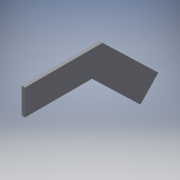
# Autodesk Inventor part: lower gusset
Saved by Autodesk Inventor 2016 (Build 200138000, 138)
## iProperties
Created: 2016-02-23
Part Number: lower gusset
Material: Aluminum 6061
Document SubType Name: Modeling
Designer: gus
Density: 2.7 g/cm^3
Appearance: Aluminum - Flat
Author: gus
Autodesk Inventor part; units mm, degrees
ref_plane "YZ Plane" through (0, 0, 0) normal (1, 0, 0) x (0, 1, 0)
ref_plane "XZ Plane" through (0, 0, 0) normal (0, 1, 0) x (-1, 0, 0)
ref_plane "XY Plane" through (0, 0, 0) normal (0, 0, 1) x (1, 0, 0)
sketch "Sketch1" plane through (0, 0, 0) normal (1, 0, 0) x (0, 1, 0)
  line L0 (0, 0) -> (0, -101.6)
  line L1 (0, -101.6) -> (-52.8555, -156.4884)
  line L2 (-25.4, 2.4125) -> (-25.4, -91.3586)
  line L3 (-25.4, -91.3586) -> (-71.1516, -138.8699)
  line L4 (-52.8555, -156.4884) -> (-71.1516, -138.8699)
  line L5 (0, 0) -> (-25.4, 0)
  dimension "d0" = 101.6
  dimension "d1" = 25.4
  dimension "d2" = 25.4
  dimension "d3" = 76.2
  dimension "d4" = 136.081
  constraints: 12 end point, 2 perpendicular, 2 vertical, 1 parallel, 1 point on line
  measures "d0" distance of L0.start L0.end
  measures "d1" distance between parallel lines of L3 L1
  measures "d2" distance between parallel lines of L2 L0
  measures "d3" distance of L0.end L1.end
  measures "d4" angle of L3 L2
extrude "Extrusion1" add sketch "Sketch1" along normal blind 3.175
body "Solid1"
